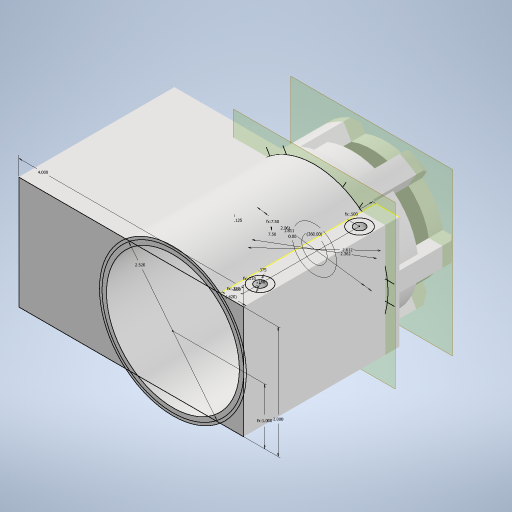
# Autodesk Inventor part: Part142
Saved by Autodesk Inventor 2023 (Build 270158000, 158)
## iProperties
Created: 2023-03-28
Part Number: Part142
Material: Generic
Document SubType Name: Modeling
Designer: Gabriel - T3 CAD
Density: 1 g/cm^3
Appearance: Default
Author: Gabriel - T3 CAD
Autodesk Inventor part; units mm, degrees
ref_plane "YZ Plane" through (0, 0, 0) normal (1, 0, 0) x (0, 1, 0)
ref_plane "XZ Plane" through (0, 0, 0) normal (0, 1, 0) x (-1, 0, 0)
ref_plane "XY Plane" through (0, 0, 0) normal (0, 0, 1) x (1, 0, 0)
sketch "Sketch1" plane through (0, 0, 0) normal (0, 0, 1) x (1, 0, 0)
  circle A0 centre (0, 0) radius 30
  circle A1 centre (0, 0) radius 33.175
  dimension "d0" = 60
  dimension "d1" = 66.35
  constraints: 3 coincident, 2 centre point
  measures "d0" diameter of A0
  measures "d1" diameter of A1
extrude "Extrusion1" add sketch "Sketch1" along normal blind 6.35
ref_plane "Work Plane1" through (0, 0, -83.5) normal (0, 0, -1) x (-1, 0, 0)
sketch "Sketch2" plane through (0, 0, -83.5) normal (0, 0, -1) x (-1, 0, 0)
  circle A0 centre (0, 0) radius 30
  circle A1 centre (0, 0) radius 33.175
  circle A2 centre (0, 0) radius 23
  circle A3 centre (0, 0) radius 26.175
  dimension "d5" = 60
  dimension "d6" = 66.35
  dimension "d28" = 46
  dimension "d29" = 52.35
  constraints: 9 coincident, 4 centre point
  measures "d5" diameter of A0
  measures "d6" diameter of A1
  measures "d28" diameter of A2
  measures "d29" diameter of A3
ref_plane "Work Plane2" through (0, 0, -57.65) normal (0, 0, -1) x (-1, 0, 0)
sketch "Sketch3" plane through (0, 0, -57.65) normal (0, 0, -1) x (-1, 0, 0)
  circle A0 centre (0, 0) radius 33.175
  circle A1 centre (0, 0) radius 30
  circle A2 centre (0, 0) radius 23
  circle A3 centre (0, 0) radius 26.175
  line L0 (0, 0) -> (33.175, 0)
  line L1 (0, 0) -> (33.175, 0) construction
  line L2 (0, 0) -> (32.8912, 4.3302)
  line L3 (0, 0) -> (32.8912, -4.3302)
  line L4 (32.8912, 4.3302) -> (32.8912, -4.3302)
  line L5 (32.8912, -4.3302) -> (0, -4.3302)
  line L6 (0, -4.3302) -> (0, 4.3302)
  line L7 (0, 4.3302) -> (32.8912, 4.3302)
  line L8 (32.8912, 4.3302) -> (32.8912, -4.3302)
  line L9 (32.8912, -4.3302) -> (36.0662, -4.3302)
  line L10 (36.0662, -4.3302) -> (36.0662, 4.3302)
  line L11 (36.0662, 4.3302) -> (32.8912, 4.3302)
  line L12 (-3.7501, 2.1651) -> (12.6955, 30.6497)
  line L13 (20.1957, 26.3195) -> (3.7501, -2.1651)
  line L14 (20.1957, 26.3195) -> (21.7832, 29.0691)
  line L15 (14.283, 33.3993) -> (12.6955, 30.6497)
  line L16 (-3.7501, -2.1651) -> (-20.1957, 26.3195)
  line L17 (-12.6955, 30.6497) -> (3.7501, 2.1651)
  line L18 (-12.6955, 30.6497) -> (-14.283, 33.3993)
  line L19 (-21.7832, 29.0691) -> (-20.1957, 26.3195)
  line L20 (0, -4.3302) -> (-32.8912, -4.3302)
  line L21 (-32.8912, 4.3302) -> (0, 4.3302)
  line L22 (-32.8912, 4.3302) -> (-36.0662, 4.3302)
  line L23 (-36.0662, -4.3302) -> (-32.8912, -4.3302)
  line L24 (3.7501, -2.1651) -> (-12.6955, -30.6497)
  line L25 (-20.1957, -26.3195) -> (-3.7501, 2.1651)
  line L26 (-20.1957, -26.3195) -> (-21.7832, -29.0691)
  line L27 (-14.283, -33.3993) -> (-12.6955, -30.6497)
  line L28 (3.7501, 2.1651) -> (20.1957, -26.3195)
  line L29 (12.6955, -30.6497) -> (-3.7501, -2.1651)
  line L30 (12.6955, -30.6497) -> (14.283, -33.3993)
  line L31 (21.7832, -29.0691) -> (20.1957, -26.3195)
  point P0 (-25.8143, 4.3302)
  point P1 (-25.8143, -4.3302)
  point P2 (-16.6572, -20.1908)
  point P3 (-9.1571, -24.521)
  point P4 (9.1571, -24.521)
  point P5 (16.6572, -20.1908)
  point P6 (25.8143, -4.3302)
  point P7 (25.8143, 4.3302)
  point P8 (16.6572, 20.1908)
  point P9 (9.1571, 24.521)
  point P10 (-16.6572, 20.1908)
  point P11 (-9.1571, 24.521)
  dimension "d8" = 66.35
  dimension "d9" = 60
  dimension "d10" = 46
  dimension "d11" = 52.35
  dimension "d12" = 0
  dimension "d13" = 7.5
  dimension "d14" = 7.5
  dimension "d15" = 3.175
  dimension "d18" = 360
  constraints: 64 end point, 10 coincident, 4 centre point, 4 parallel, 3 point on circle, 2 perpendicular, 1 collinear, 1 horizontal, 1 midpoint, 61 other
  measures "d8" diameter of A0
  measures "d9" diameter of A1
  measures "d10" diameter of A2
  measures "d11" diameter of A3
  measures "d12" distance between parallel lines of L0 L1
  measures "d13" angle of L0 L3
  measures "d14" angle of L0 L2
  measures "d15" distance of L9.end L3.end
extrude "Extrusion2" add sketch "Sketch3" against normal up to surface (57.65 mm away) contours L0 L4 A0 | A0 L4 L0 | L7 A1 L13 A0 | L4 L0 A1 L2 | L2 A1 L7 | L5 A1 L3 | L3 A1 L0 L4 | A0 L28 A1 L5 | L13 A1 L12 A0 | A0 L29 A1 L28 | L12 A1 L17 A0 | A0 L24 A1 L29 | L17 A1 L16 A0 | A0 L25 A1 L24 | L16 A1 L21 A0 | A0 L20 A1 L25 | L21 A1 L20 A0
extrude "Extrusion3" add sketch "Sketch3" along normal blind 17 contours L2 A3 L7 A1 | A1 L0 A3 L2 | L7 A3 L13 A1 | L3 A3 L0 A1 | A1 L5 A3 L3 | A1 L28 A3 L5 | L13 A3 L12 A1 | L2 A2 L7 A3 | A3 L0 A2 L2 | L7 A2 L13 A3 | A1 L29 A3 L28 | L3 A2 L0 A3 | A3 L5 A2 L3 | A3 L28 A2 L5 | L12 A3 L17 A1 | L13 A2 L12 A3 | A1 L24 A3 L29 | A3 L29 A2 L28 | L17 A3 L16 A1 | L12 A2 L17 A3 | A1 L25 A3 L24 | A3 L24 A2 L29 | L16 A3 L21 A1 | L17 A2 L16 A3 | A1 L20 A3 L25 | A3 L25 A2 L24 | L21 A3 L20 A1 | L16 A2 L21 A3 | A3 L20 A2 L25 | L21 A2 L20 A3
extrude "Extrusion5" add sketch "Sketch3" along normal blind 6.35 contours L0 L4 A0 | A0 L4 L0 | L7 A1 L13 A0 | L4 L0 A1 L2 | L2 A1 L7 | L5 A1 L3 | L3 A1 L0 L4 | A0 L28 A1 L5 | L13 A1 L12 A0 | A0 L29 A1 L28 | L12 A1 L17 A0 | A0 L24 A1 L29 | L17 A1 L16 A0 | A0 L25 A1 L24 | L16 A1 L21 A0 | A0 L20 A1 L25 | L21 A1 L20 A0
extrude "Extrusion6" add sketch "Sketch2" along normal blind 6.35 contours A2 | A3
extrude "Extrusion4" add sketch "Sketch3" along normal up to surface (32.2 mm away) contours L0 L4 A0 | A0 L4 L0 | L4 L0 A1 L2 | L2 A1 L7 | L5 A1 L3 | L3 A1 L0 L4 | L13 A1 L12 A0 | L2 A3 L7 A1 | A1 L0 A3 L2 | A0 L29 A1 L28 | L3 A3 L0 A1 | A1 L5 A3 L3 | L13 A3 L12 A1 | A1 L29 A3 L28 | L17 A1 L16 A0 | A0 L25 A1 L24 | L17 A3 L16 A1 | A1 L25 A3 L24 | L21 A1 L20 A0 | L21 A3 L20 A1
chamfer "Chamfer1" distance 3.175 angle 45 6 edges at (16.5875, 28.7304, -89.85) (-16.5875, 28.7304, -89.85) (33.175, 0, -89.85) (16.5875, -28.7304, -89.85) (-16.5875, -28.7304, -89.85) (-33.175, 0, -89.85)
sketch "Sketch4" plane through (0, 0, 6.35) normal (0, 0, 1) x (1, 0, 0)
  circle A0 centre (0, 0) radius 32
  line L0 (32, 25.4) -> (32, -25.4)
  line L1 (32, -25.4) -> (-69.6, -25.4)
  line L2 (-69.6, -25.4) -> (-69.6, 25.4)
  line L3 (-69.6, 25.4) -> (32, 25.4)
  circle A1 centre (0, 0) radius 30
  circle A2 centre (0, 0) radius 30 projected
  circle A3 centre (0, 0) radius 33.175
  circle A4 centre (0, 0) radius 33.175 projected
  point P0 (21.3406, 25.4)
  point P1 (-21.3406, 25.4)
  point P2 (-21.3406, -25.4)
  point P3 (21.3406, -25.4)
  point P4 (32, 8.751)
  point P5 (32, -8.751)
  dimension "d41" = 64
  dimension "d42" = 25.4
  dimension "d43" = 50.8
  dimension "d44" = 101.6
  constraints: 8 end point, 3 centre point, 3 coincident, 2 concentric, 2 parallel, 1 horizontal, 1 perpendicular, 1 tangent
  measures "d41" diameter of A0
  measures "d42" distance from line of L1 point (0, 0)
  measures "d43" distance of L0.start L0.end
  measures "d44" distance of L2.end L0.start
extrude "Extrusion7" add sketch "Sketch4" against normal up to surface (70.35 mm away) contours A0 L1 A1 L3 | L0 A3 L1 A0 | A0 L3 A3 L0 | L3 A1 A0 | A0 L3 A3 | L1 A3 A0 | A0 L1 A1 | A3 L3 L0 | L0 L1 A3 | L3 A1 L1 A0 | A0 L1 A3 L3 | A3 L1 L2 L3
extrude "Extrusion8" cut sketch "Sketch4" against normal through all contours L0 A3
sketch "Sketch7" plane through (21.3406, 25.4, 6.35) normal (0, 1, 0) x (1, 0, 0)
  circle A0 centre (5.3297, 12.7) radius 2.3813
  circle A1 centre (5.3297, 57.65) radius 2.3813
  line L0 (0, 0) -> (0, 70.35) projected
  line L1 (10.6594, 0) -> (0, 0) projected
  line L2 (10.6594, 70.35) -> (0, 70.35) projected
  circle A2 centre (5.3297, 12.7) radius 4.7625
  circle A3 centre (5.3297, 57.65) radius 4.7625
  point P0 (-21.3406, 6.35)
  dimension "d67" = 4.7625
  dimension "d68" = 5.3297
  dimension "d69" = 5.3297
  dimension "d70" = 12.7
  dimension "d71" = 12.7
  dimension "d72" = 10.6594
  dimension "d73" = 9.525
  constraints: 4 centre point, 2 coincident, 2 equal radius
  measures "d67" diameter of A0
  measures "d68" distance from line of L0 A0.centre
  measures "d69" distance from line of L0 A1.centre
  measures "d70" distance from line of A0.centre L1
  measures "d71" distance from line of L2 A1.centre
  measures "d72" distance of L1.start L0.start
  measures "d73" diameter of A2
extrude "Extrusion11" cut sketch "Sketch7" against normal blind 6.35 contours A0 | A1 | A2 | A3
extrude "Extrusion12" add sketch "Sketch7" against normal blind 1.5875
equation "\"d14\" = d13"
equation "\"d42\" = 0.5 * d43"
equation "\"d68\" = 0.5 * d72"
equation "\"d69\" = d68"
equation "\"d71\" = d70"
body "Solid1"
